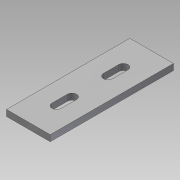
# Autodesk Inventor part: StairsConnectionPlate
Saved by Autodesk Inventor 2015 (Build 190159000, 159)
## iProperties
Created: 2015-03-25
Part Number: StairsConnectionPlate
Material: Steel
Document SubType Name: Modeling
Designer: m_crauwels
Density: 7.85 g/cm^3
Appearance: Steel
Mass: 1772 g
Surface Area: 482.193 cm^2
Volume: 225.733 cm^3
d42: 85.000 mm
d43: 240.000 mm
d44: 12.000 mm
d45: 0.00 deg
d46: 100.000 mm
d47: 30.000 mm
d48: 18.000 mm
d49: 30.000 mm
d50: 18.000 mm
d51: 0.00 deg
Author: m_crauwels
Autodesk Inventor part; units mm, degrees
ref_plane "YZ Plane" through (0, 0, 0) normal (1, 0, 0) x (0, 1, 0)
ref_plane "XZ Plane" through (0, 0, 0) normal (0, 1, 0) x (-1, 0, 0)
ref_plane "XY Plane" through (0, 0, 0) normal (0, 0, 1) x (1, 0, 0)
sketch "Sketch1" plane through (0, 0, 0) normal (0, 0, 1) x (1, 0, 0)
  line L0 (42.5, -120) -> (-42.5, -120)
  line L1 (-42.5, -120) -> (-42.5, 120)
  line L2 (-42.5, 120) -> (42.5, 120)
  line L3 (42.5, 120) -> (42.5, -120)
  line L4 (42.5, -120) -> (-42.5, 120) construction
  line L5 (-42.5, -120) -> (42.5, 120) construction
  point P0 (0, 0)
  dimension "d42" = 85
  dimension "d43" = 240
  constraints: 12 end point, 2 midpoint, 2 parallel, 1 horizontal, 1 perpendicular
  measures "d42" distance of L1.end L2.end
  measures "d43" distance of L0.end L1.end
extrude "Extrusion1" add sketch "Sketch1" against normal blind 12
sketch "Sketch2" plane through (0, 0, -12) normal (0, 0, -1) x (1, 0, 0)
  line L0 (42.5, -120) -> (42.5, 120) projected
  line L1 (0, -50) -> (0, 50)
  line L2 (0, -65) -> (0, -35) construction
  line L3 (9, -65) -> (9, -35)
  line L4 (-9, -35) -> (-9, -65)
  arc A0 (-9, -65) -> (9, -65) centre (0, -65) ccw
  arc A1 (9, -35) -> (-9, -35) centre (0, -35) ccw
  line L5 (0, 35) -> (0, 65) construction
  line L6 (9, 35) -> (9, 65)
  line L7 (-9, 65) -> (-9, 35)
  arc A2 (-9, 35) -> (9, 35) centre (0, 35) ccw
  arc A3 (9, 65) -> (-9, 65) centre (0, 65) ccw
  point P0 (0, 0)
  point P1 (0, -50)
  point P2 (0, 0)
  dimension "d46" = 100
  dimension "d47" = 30
  dimension "d48" = 18
  dimension "d49" = 30
  dimension "d50" = 18
  constraints: 18 end point, 8 point on circle, 8 tangent, 4 centre point, 4 parallel, 3 coincident, 3 midpoint, 1 vertical
  measures "d46" distance of L1.start L1.end
  measures "d47" distance of L2.start L2.end
  measures "d48" diameter of A1
  measures "d49" distance of L5.start L5.end
  measures "d50" diameter of A3
extrude "Extrusion2" cut sketch "Sketch2" against normal through all
equation "\"d49\" = d47"
equation "\"d50\" = d48"
body "Solid1"
